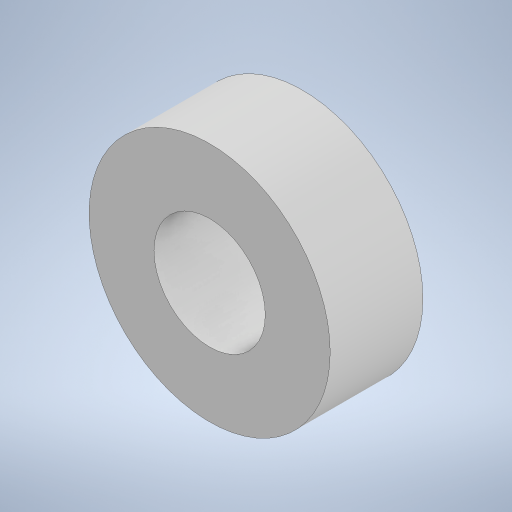
# Autodesk Inventor part: Housing
Saved by Autodesk Inventor 2023 (Build 270158000, 158)
## iProperties
Created: 2023-01-17
Part Number: Housing
Material: Generic
Document SubType Name: Modeling
Designer: caden
Density: 1 g/cm^3
Appearance: Default
Description: 3D Print
Author: caden
Autodesk Inventor part; units mm, degrees
ref_plane "YZ Plane" through (0, 0, 0) normal (1, 0, 0) x (0, 1, 0)
ref_plane "XZ Plane" through (0, 0, 0) normal (0, 1, 0) x (-1, 0, 0)
ref_plane "XY Plane" through (0, 0, 0) normal (0, 0, 1) x (1, 0, 0)
sketch "Sketch1" plane through (0, 0, 0) normal (0, 0, 1) x (1, 0, 0)
  circle A0 centre (0, 0) radius 60 construction
  circle A1 centre (-60, 0) radius 6.5
  dimension "d5" = 120
  dimension "d0" = 13
  constraints: 1 centre point, 1 coincident, 1 horizontal alignment, 2 other
  measures "d0" diameter of A1
extrude "Extrusion1" add sketch "Sketch1" along normal blind 5
sketch "Sketch2" plane through (-60, 0, 5) normal (0, 0, 1) x (1, 0, 0)
  circle A0 centre (60, 0) radius 60 construction
  circle A1 centre (0, 0) radius 6.5 projected
  circle A2 centre (0, 0) radius 3
  circle A3 centre (2.6656, -17.6853) radius 3
  circle A4 centre (10.4257, -33.7992) radius 3
  circle A5 centre (22.5906, -46.9099) radius 3
  circle A6 centre (38.0795, -55.8524) radius 3
  circle A7 centre (55.5162, -59.8322) radius 3
  circle A8 centre (73.3513, -58.4957) radius 3
  circle A9 centre (90, -51.9615) radius 3
  circle A10 centre (103.9831, -40.8104) radius 3
  circle A11 centre (114.0581, -26.033) radius 3
  circle A12 centre (119.3298, -8.9425) radius 3
  circle A13 centre (119.3298, 8.9425) radius 3
  circle A14 centre (114.0581, 26.033) radius 3
  circle A15 centre (103.9831, 40.8104) radius 3
  circle A16 centre (90, 51.9615) radius 3
  circle A17 centre (73.3513, 58.4957) radius 3
  circle A18 centre (55.5162, 59.8322) radius 3
  circle A19 centre (38.0795, 55.8524) radius 3
  circle A20 centre (22.5906, 46.9099) radius 3
  circle A21 centre (10.4257, 33.7992) radius 3
  circle A22 centre (2.6656, 17.6853) radius 3
  dimension "d8" = 120
  dimension "d9" = 6
  dimension "d12" = 360
  constraints: 22 centre point, 2 coincident, 43 other
  measures "d8" diameter of A0
  measures "d9" diameter of A2
extrude "Extrusion2" cut sketch "Sketch2" against normal through all contours A2 | A3 | A4 | A5 | A6 | A7 | A8 | A9 | A10 | A11 | A12 | A13 | A14 | A15 | A16 | A17 | A18 | A19 | A20 | A21 | A22
body "Solid1"
